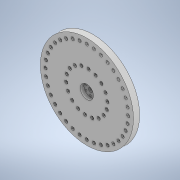
# Autodesk Inventor part: front_plate
Saved by Autodesk Inventor 2020.3 (Build 243373000, 373)
## iProperties
Created: 2020-11-01
Part Number: front_plate
Material: Generic
Document SubType Name: Modeling
Designer: Martijn
Density: 1 g/cm^3
Appearance: Default
Author: Martijn
Autodesk Inventor part; units mm, degrees
ref_plane "YZ Plane" through (0, 0, 0) normal (1, 0, 0) x (0, 1, 0)
ref_plane "XZ Plane" through (0, 0, 0) normal (0, 1, 0) x (-1, 0, 0)
ref_plane "XY Plane" through (0, 0, 0) normal (0, 0, 1) x (1, 0, 0)
sketch "Sketch1" plane through (0, 0, 0) normal (0, 0, 1) x (1, 0, 0)
  circle A0 centre (0, 0) radius 90
  dimension "d2" = 180
  constraints: 1 centre point, 1 coincident
  measures "d2" diameter of A0
extrude "Extrusion1" add sketch "Sketch1" along normal blind 5
sketch "Sketch2" plane through (0, 0, 5) normal (0, 0, 1) x (1, 0, 0)
  circle A0 centre (0, 0) radius 90
  circle A1 centre (0, 0) radius 90 projected
  circle A2 centre (0, 0) radius 12.8
  dimension "d3" = 25.6
  constraints: 2 centre point, 2 coincident, 1 concentric
  measures "d3" diameter of A2
extrude "Extrusion2" add sketch "Sketch2" along normal blind 7
sketch "Sketch4" plane through (0, 0, 5) normal (0, 0, 1) x (1, 0, 0)
  circle A0 centre (0, 0) radius 4
  dimension "d13" = 8
  constraints: 1 centre point, 1 coincident
  measures "d13" diameter of A0
extrude "Extrusion4" cut sketch "Sketch4" against normal blind 7
sketch "Sketch3" plane through (0, 0, 5) normal (0, 0, 1) x (1, 0, 0)
  circle A0 centre (0, 9.525) radius 1.6
  line L0 (0, -126) -> (0, 126) projected
  point P0 (0, 0)
  dimension "d6" = 3.2
  dimension "d7" = 9.525
  constraints: 1 centre point, 1 point on line
  measures "d6" diameter of A0
  measures "d7" distance of point (0, 0) A0.centre
extrude "Extrusion3" cut sketch "Sketch3" against normal blind 10
pattern_circular "Circular Pattern2" count 6 over 360 about axis through (0, 0, 5) along (0, 0, 1) of "Extrusion3"
sketch "Sketch7" plane through (0, 0, 12) normal (0, 0, 1) x (1, 0, 0)
  circle A0 centre (0, 80) radius 1.6
  circle A1 centre (13.8919, 78.7846) radius 1.6
  line L0 (13.8919, 78.7846) -> (0, 0)
  line L1 (0, 80) -> (0, 0)
  circle A2 centre (3.4862, 39.8478) radius 1.6
  line L2 (3.4862, 39.8478) -> (0, 0)
  dimension "d22" = 3.2
  dimension "d23" = 80
  dimension "d24" = 80
  dimension "d25" = 10
  dimension "d26" = 40
  dimension "d27" = 5
  dimension "d28" = 3.2
  dimension "d29" = 3.2
  constraints: 6 end point, 3 centre point, 1 vertical
  measures "d22" diameter of A0
  measures "d23" distance of L0.end L1.start
  measures "d24" distance of L0.start L0.end
  measures "d25" angle of L1 L0
  measures "d26" distance of L2.start L0.end
  measures "d27" angle of L0 L2
  measures "d28" diameter of A2
  measures "d29" diameter of A1
extrude "Extrusion6" cut sketch "Sketch7" against normal through all
sketch "Sketch8" plane through (0, 0, 12) normal (0, 0, 1) x (1, 0, 0)
  line L0 (-1.6454, 82.85) -> (1.6454, 82.85)
  line L1 (1.6454, 82.85) -> (3.2909, 80)
  line L2 (3.2909, 80) -> (1.6454, 77.15)
  line L3 (1.6454, 77.15) -> (-1.6454, 77.15)
  line L4 (-1.6454, 77.15) -> (-3.2909, 80)
  line L5 (-3.2909, 80) -> (-1.6454, 82.85)
  line L6 (-1.6454, 82.85) -> (1.6454, 77.15)
  line L7 (12.7663, 81.8771) -> (16.0072, 81.3056)
  line L8 (16.0072, 81.3056) -> (17.1328, 78.2132)
  line L9 (17.1328, 78.2132) -> (15.0174, 75.6922)
  line L10 (15.0174, 75.6922) -> (11.7765, 76.2636)
  line L11 (11.7765, 76.2636) -> (10.651, 79.3561)
  line L12 (10.651, 79.3561) -> (12.7663, 81.8771)
  line L13 (12.7663, 81.8771) -> (15.0174, 75.6922)
  circle A0 centre (13.8919, 78.7846) radius 1.6
  circle A1 centre (13.8919, 78.7846) radius 1.6 projected
  line L14 (2.0954, 42.8304) -> (5.3738, 42.5435)
  line L15 (5.3738, 42.5435) -> (6.7646, 39.561)
  line L16 (6.7646, 39.561) -> (4.877, 36.8652)
  line L17 (4.877, 36.8652) -> (1.5986, 37.152)
  line L18 (1.5986, 37.152) -> (0.2079, 40.1346)
  line L19 (0.2079, 40.1346) -> (2.0954, 42.8304)
  line L20 (2.0954, 42.8304) -> (4.877, 36.8652)
  circle A2 centre (3.4862, 39.8478) radius 1.6 projected
  circle A3 centre (3.4862, 39.8478) radius 1.6
  circle A4 centre (3.4862, 39.8478) radius 1.6 projected
  circle A5 centre (0, 80) radius 1.6
  circle A6 centre (0, 80) radius 1.6 projected
  point P0 (0, 0)
  dimension "d33" = 5.7
  dimension "d34" = 120
  dimension "d35" = 120
  dimension "d36" = 120
  dimension "d37" = 120
  dimension "d38" = 5.7
  dimension "d39" = 170
  dimension "d40" = 120
  dimension "d41" = 120
  dimension "d42" = 5.7
  dimension "d43" = 5
  constraints: 42 end point, 12 equal length, 6 concentric, 6 parallel, 5 coincident, 3 centre point, 3 midpoint, 1 horizontal
  measures "d33" distance between parallel lines of L3 L0
  measures "d34" angle of L3 L4
  measures "d35" angle of L4 L5
  measures "d36" angle of L12 L7
  measures "d37" angle of L11 L12
  measures "d38" distance between parallel lines of L10 L7
  measures "d39" angle of L10 L3
  measures "d40" angle of L18 L19
  measures "d41" angle of L19 L14
  measures "d42" distance between parallel lines of L17 L14
  measures "d43" angle of L3 L17
extrude "Extrusion7" cut sketch "Sketch8" against normal blind 7 contours L6 A5 L3 L4 L5 | L0 L1 L2 L6 A5 | A5 L6 | L6 A5 | L13 A0 L10 L11 L12 | L7 L8 L9 L13 A0 | L20 A2 L17 L18 L19 | L14 L15 L16 L20 A2
pattern_circular "Circular Pattern3" count 18 over 360 about axis through (0, 0, 0) along (0, 0, 1) of "Extrusion7", "Extrusion6"
body "Solid1"
